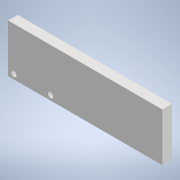
# Autodesk Inventor part: Part18
Saved by Autodesk Inventor 2020.2 (Build 242310000, 310)
## iProperties
Created: 2022-11-15
Part Number: Part18
Material: 一般
Document SubType Name: Modeling
Designer: Administrator
Density: 1 g/cm^3
Appearance: 既定
Author: Administrator
Autodesk Inventor part; units mm, degrees
ref_plane "YZ Plane" through (0, 0, 0) normal (1, 0, 0) x (0, 1, 0)
ref_plane "XZ Plane" through (0, 0, 0) normal (0, 1, 0) x (-1, 0, 0)
ref_plane "XY Plane" through (0, 0, 0) normal (0, 0, 1) x (1, 0, 0)
sketch "スケッチ1" plane through (0, 0, 0) normal (0, 0, 1) x (1, 0, 0)
  line L0 (34.5, -2.7) -> (15.5, -2.7) projected
  line L1 (50, -5) -> (0, -5) projected
  line L2 (12, -5) -> (12, 5) projected
  circle A0 centre (44, 0) radius 2.75 projected
  circle A1 centre (6, 0) radius 2.75 projected
  line L3 (50, -5) -> (50, 5) projected
  line L4 (0, 5) -> (50, 5) projected
  line L5 (0, -5) -> (0, 5) projected
  line L6 (50, -5) -> (0, -5) projected
  line L7 (0, -5) -> (160, -5)
  line L8 (160, -5) -> (160, 45)
  line L9 (160, 45) -> (0, 45)
  line L10 (0, 45) -> (0, -5)
  point P0 (0, 0)
  dimension "d0" = 160
  dimension "d1" = 50
  constraints: 8 end point, 2 parallel, 1 horizontal, 1 perpendicular
  measures "d0" distance of L9.end L8.end
  measures "d1" distance of L8.end L7.end
extrude "押し出し1" add sketch "スケッチ1" along normal blind 10
